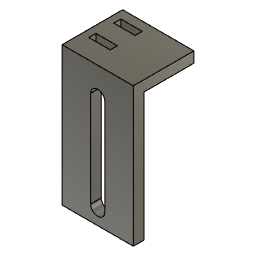
wire_guide_TOP v3 (Autodesk Fusion 360 design; units mm, degrees)
Autodesk Fusion 360 part; units mm, degrees
sketch "Sketch1" plane through (0, 0, 0) normal (0, 1, 0) x (1, 0, 0)
  line L0 (0, 0) -> (10, 0)
  line L1 (10, 0) -> (10, -59.85)
  line L2 (10, -59.85) -> (0, -59.85)
  line L3 (0, -59.85) -> (0, 0)
  dimension "d1" = 10
  dimension "d2" = 59.85
  constraint horizontal L0
  constraint vertical L1
  constraint horizontal L2
  constraint vertical L3
  constraint coincident L0.start L3.end
  measures "d1" distance of L0.start L0.end
  measures "d2" distance of L0.start L2.end
extrude "Extrude1" add sketch "Sketch1" along normal blind 3
sketch "Sketch2" plane through (0, 0, 59.85) normal (0, 0, 1) x (-1, 0, 0)
  line L0 (0, 0) -> (-10, 0)
  line L1 (-10, 0) -> (-10, -3)
  line L2 (-10, -3) -> (0, -3)
  line L3 (0, -3) -> (0, 0)
  line L4 (0, 0) -> (-10, 0)
  line L5 (-10, 0) -> (-10, -17)
  line L6 (-10, -17) -> (0, -17)
  line L7 (0, -17) -> (0, 0)
  dimension "d5" = 17
  constraint horizontal L4
  constraint vertical L5
  constraint horizontal L6
  constraint vertical L7
  constraint coincident L0.start L3.end
  measures "d5" distance of L0.start L6.end
extrude "Extrude2" add sketch "Sketch2" along normal blind 3
sketch "Sketch3" plane through (0, 0, 62.85) normal (0, 0, 1) x (-1, 0, 0)
  line L0 (0, -17) -> (0, 0)
  line L1 (0, 0) -> (-10, 0)
  line L2 (-10, 0) -> (-10, -17)
  line L3 (-10, -17) -> (0, -17)
  line L4 (0, -3) -> (-10, -3)
  line L5 (-5, -17) -> (-5, -3) construction
  line L6 (-5, -10) -> (-5, -12.5)
  line L7 (-5, -10) -> (-5, -7.5)
  line L8 (-5, -7.5) -> (-2, -7.5)
  line L9 (-2, -7.5) -> (-2, -5.5)
  line L10 (-2, -5.5) -> (-5, -5.5)
  line L11 (-5, -5.5) -> (-5, -7.5)
  line L12 (-5, -7.5) -> (-8, -7.5)
  line L13 (-8, -7.5) -> (-8, -5.5)
  line L14 (-8, -5.5) -> (-5, -5.5)
  line L15 (-5, -10) -> (-2.0194, -10) construction
  line L16 (-5, -12.5) -> (-2, -12.5)
  line L17 (-2, -12.5) -> (-2, -14.5)
  line L18 (-2, -14.5) -> (-5, -14.5)
  line L19 (-8, -14.5) -> (-5, -14.5)
  line L20 (-8, -12.5) -> (-8, -14.5)
  line L21 (-5, -12.5) -> (-8, -12.5)
  dimension "d8" = 2.5
  dimension "d9" = 2.5
  dimension "d10" = 3
  dimension "d11" = 2
  constraint midpoint L3 L5.start
  constraint midpoint L4 L5.end
  constraint midpoint L5 L6.start
  constraint parallel L5 L6
  constraint parallel L5 L7
  constraint horizontal L8
  constraint vertical L9
  constraint horizontal L10
  constraint vertical L11
  constraint symmetric L7.end L11 L8.start
  constraint symmetric L8.end L11 L12.end
  constraint symmetric L9.end L11 L13.end
  constraint symmetric L10.end L11 L14.end
  constraint perpendicular L5 L15
  constraint symmetric L7.end L15 L6.end
  constraint symmetric L8.end L15 L16.end
  constraint symmetric L9.end L15 L17.end
  constraint symmetric L10.end L15 L18.end
  constraint symmetric L12.end L15 L20.start
  constraint symmetric L13.end L15 L19.start
  measures "d8" distance of L6.start L6.end
  measures "d9" distance of L6.start L7.end
  measures "d10" distance of L7.end L8.end
  measures "d11" distance of L7.end L10.end
extrude "Extrude3" cut sketch "Sketch3" against normal up to surface (3 mm away) contours L8 L9 L10 L11 | L11 L12 L13 L14 | L16 L17 L18 L19 L20 L21
sketch "Sketch4" plane through (0, 0, 0) normal (0, 0, -1) x (1, 0, 0)
  line L0 (10, 0) -> (0, 0)
  line L1 (0, 0) -> (0, -3)
  line L2 (0, -3) -> (10, -3)
  line L3 (10, -3) -> (10, 0)
  line L4 (0, -3) -> (10, -3)
  line L5 (10, -3) -> (10, 14)
  line L6 (10, 14) -> (0, 14)
  line L7 (0, 14) -> (0, -3)
  line L8 (5, 14) -> (5, 0) construction
  line L9 (0, 14) -> (0, 7)
  line L10 (0, 7) -> (10, 7) construction
  circle A0 centre (5, 7) radius 2
  dimension "d14" = 17
  dimension "d15" = 7
  dimension "d16" = 4
  constraint horizontal L4
  constraint vertical L5
  constraint horizontal L6
  constraint vertical L7
  constraint coincident L1.end L2.start
  constraint midpoint L6 L8.start
  constraint midpoint L0 L8.end
  constraint perpendicular L0 L8
  constraint perpendicular L6 L9
  constraint coincident L5 L10.end
  constraint perpendicular L5 L10
  constraint midpoint L10 A0.centre
  measures "d14" distance of L1.end L6.end
  measures "d15" distance of L6.end L9.end
  measures "d16" diameter of A0
extrude "Extrude4" add sketch "Sketch4" against normal blind 3 contours L0 L5 L6 L7 L9
move_face "OffsetFaces1" offset 10 1 faces at (10, 2, 20.95)
sketch "Sketch5" plane through (0, 0, 3) normal (0, 0, 1) x (-1, 0, 0)
  circle A0 centre (-5, 7) radius 2
  line L0 (-20, 14) -> (-20, 0)
  line L1 (-20, 0) -> (0, 0)
  line L2 (0, 0) -> (0, 14)
  line L3 (0, 14) -> (-20, 14)
  line L4 (-10, 14) -> (-10, 0) construction
  circle A1 centre (-15, 7) radius 2
  constraint midpoint L3 L4.start
  constraint midpoint L1 L4.end
  constraint symmetric A0 L4 A1
extrude "Extrude5" cut sketch "Sketch5" against normal up to surface (3 mm away) contours A1
sketch "Sketch6" plane through (0, 0, 0) normal (0, 0, -1) x (1, 0, 0)
  circle A0 centre (15, 7) radius 2
  circle A1 centre (5, 7) radius 2
  line L0 (0, 14) -> (0, -3)
  line L1 (0, -3) -> (20, -3)
  line L2 (20, -3) -> (20, 14)
  line L3 (20, 14) -> (0, 14)
  line L4 (-9.2754, 20.5628) -> (28.3426, 20.5628)
  line L5 (28.3426, 20.5628) -> (28.3426, -10.0286)
  line L6 (28.3426, -10.0286) -> (-9.2754, -10.0286)
  line L7 (-9.2754, -10.0286) -> (-9.2754, 20.5628)
  constraint horizontal L4
  constraint vertical L5
  constraint horizontal L6
  constraint vertical L7
extrude "Extrude6" cut sketch "Sketch6" against normal blind 9.85 contours L0 L1 L2 L3 | L4 L5 L6 L7
sketch "Sketch8" plane through (0, 0, 9.85) normal (0, 0, -1) x (1, 0, 0)
  line L0 (20, -3) -> (20, 0)
  line L1 (20, 0) -> (0, 0)
  line L2 (0, 0) -> (0, -3)
  line L3 (0, -3) -> (20, -3)
  line L4 (0, -3) -> (20, -3)
  line L5 (20, -3) -> (20, 14)
  line L6 (20, 14) -> (0, 14)
  line L7 (0, 14) -> (0, -3)
  line L8 (10, 14) -> (10, -3)
  line L9 (0, 5.9968) -> (10, 5.9968)
  circle A0 centre (5, 5.9968) radius 2
  circle A1 centre (15, 5.9968) radius 2
  dimension "d29" = 17
  dimension "d30" = 4
  constraint horizontal L4
  constraint vertical L5
  constraint horizontal L6
  constraint vertical L7
  constraint coincident L2.end L3.start
  constraint midpoint L6 L8.start
  constraint midpoint L4 L8.end
  constraint coincident L7 L9.start
  constraint coincident L8 L9.end
  constraint perpendicular L8 L9
  constraint midpoint L9 A0.centre
  constraint symmetric L8 A0 A1
  measures "d29" distance of L2.end L6.end
  measures "d30" diameter of A0
extrude "Extrude8" add sketch "Sketch8" along normal blind 3 contours L0 L1 L3 L4 L5 L8 | L1 L5 L6 L8 | L1 L2 L3 L4 L7 L8 | L1 L7 L8 L9 A0 | L6 L7 L8 L9 A0
sketch "Sketch9" plane through (0, 0, 0) normal (0, -1, 0) x (1, 0, 0)
  line L0 (0, 9.85) -> (20, 9.85)
  line L1 (20, 9.85) -> (20, 62.85)
  line L2 (20, 62.85) -> (0, 62.85)
  line L3 (0, 62.85) -> (0, 9.85)
  line L4 (10, 62.85) -> (10, 9.85) construction
  circle A0 centre (10, 55.0319) radius 2
  circle A1 centre (10, 28.1174) radius 2
  line L5 (8, 55.032) -> (8, 28.1174)
  line L6 (12, 55.032) -> (12, 28.1174)
  dimension "d33" = 4
  dimension "d34" = 4
  constraint midpoint L2 L4.start
  constraint midpoint L0 L4.end
  constraint coincident L4 A0.centre
  constraint coincident L4 A1.centre
  constraint coincident A0 L5.start
  constraint coincident A1 L5.end
  constraint tangent A1 L5
  constraint parallel L4 L5
  constraint coincident A0 L6.start
  constraint coincident A1 L6.end
  constraint tangent A1 L6
  constraint parallel L4 L6
  measures "d33" diameter of A0
  measures "d34" diameter of A1
extrude "Extrude9" cut sketch "Sketch9" against normal blind 3 contours A0 | A0 A1 L5 L6 | A1
sketch "Sketch10" plane through (0, 0, 6.85) normal (0, 0, -1) x (1, 0, 0)
  circle A0 centre (5, 5.9968) radius 2
  circle A1 centre (15, 5.9968) radius 2
  line L0 (0, 14) -> (0, -3)
  line L1 (0, -3) -> (20, -3)
  line L2 (20, -3) -> (20, 14)
  line L3 (20, 14) -> (0, 14)
  line L4 (-4.2191, 16.8047) -> (27.4673, 16.8047)
  line L5 (27.4673, 16.8047) -> (27.4673, -8.4841)
  line L6 (27.4673, -8.4841) -> (-4.2191, -8.4841)
  line L7 (-4.2191, -8.4841) -> (-4.2191, 16.8047)
  constraint horizontal L4
  constraint vertical L5
  constraint horizontal L6
  constraint vertical L7
extrude "Extrude10" cut sketch "Sketch10" against normal blind 17 contours L0 L1 L2 L3 | L4 L5 L6 L7
